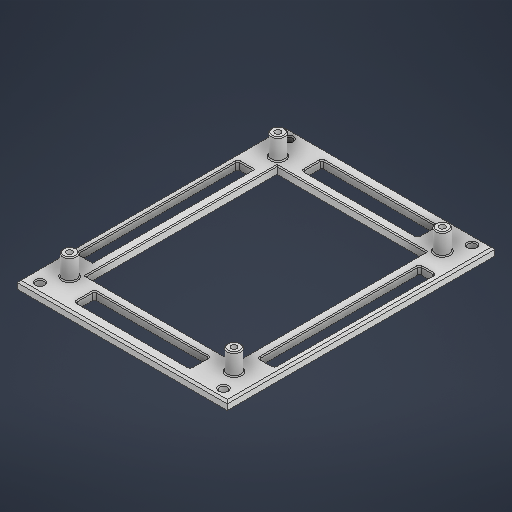
# Autodesk Inventor part: Base
Saved by Autodesk Inventor 2026 (Build 300175000, 175)
## iProperties
Created: 2026-02-15
Part Number: Base
Material: Generisch
Document SubType Name: Modeling
Designer: Jakob Dorninger
Density: 1 g/cm^3
Appearance: Vorgabe
Author: Jakob Dorninger
Autodesk Inventor part; units mm, degrees
ref_plane "YZ Plane" through (0, 0, 0) normal (1, 0, 0) x (0, 1, 0)
ref_plane "XZ Plane" through (0, 0, 0) normal (0, 1, 0) x (-1, 0, 0)
ref_plane "XY Plane" through (0, 0, 0) normal (0, 0, 1) x (1, 0, 0)
sketch "Skizze1" plane through (0, 0, 0) normal (0, 0, 1) x (1, 0, 0)
  line L0 (27.5, -35) -> (-27.5, -35)
  line L1 (-27.5, -35) -> (-27.5, 35)
  line L2 (-27.5, 35) -> (27.5, 35)
  line L3 (27.5, 35) -> (27.5, -35)
  line L4 (27.5, -35) -> (-27.5, 35) construction
  line L5 (-27.5, -35) -> (27.5, 35) construction
  line L6 (-19.5, -25) -> (19.5, -25)
  line L7 (19.5, -25) -> (19.5, 25)
  line L8 (19.5, 25) -> (-19.5, 25)
  line L9 (-19.5, 25) -> (-19.5, -25)
  line L10 (-19.5, -25) -> (19.5, 25) construction
  line L11 (19.5, -25) -> (-19.5, 25) construction
  point P0 (0, 0)
  dimension "d0" = 55
  dimension "d1" = 70
  dimension "d32" = 39
  dimension "d33" = 50
  constraints: 24 end point, 4 midpoint, 4 parallel, 2 horizontal, 2 perpendicular
  measures "d0" distance of L1.end L2.end
  measures "d1" distance of L0.end L1.end
  measures "d32" distance of L8.end L7.end
  measures "d33" distance of L7.end L6.end
extrude "Extrusion1" add sketch "Skizze1" along normal blind 2
sketch "Skizze2" plane through (0, 0, 2) normal (0, 0, 1) x (1, 0, 0)
  circle A0 centre (-21.5, 27.25) radius 1.75
  line L0 (0, -49) -> (0, 49) projected
  line L1 (-38.5, 0) -> (38.5, 0) projected
  circle A1 centre (-21.5, -27.25) radius 1.75
  circle A2 centre (21.5, 27.25) radius 1.75
  circle A3 centre (21.5, -27.25) radius 1.75
  point P0 (0, 0)
  dimension "d4" = 3.5
  dimension "d5" = 21.5
  dimension "d6" = 27.25
  dimension "d9" = 54.5
  dimension "d12" = 43
  constraints: 4 centre point, 1 horizontal, 1 vertical, 6 other
  measures "d4" diameter of A0
  measures "d5" horizontal distance of point (0, 0) A0.centre
  measures "d6" vertical distance of point (0, 0) A0.centre
  measures "d9" distance of A0.centre A1.centre
  measures "d12" distance of A0.centre A2.centre
extrude "Extrusion2" add sketch "Skizze2" along normal blind 5.5
sketch "Skizze3" plane through (-21.5, 27.25, 7.5) normal (0, 0, 1) x (1, 0, 0)
  circle A0 centre (0, 0) radius 1.75 projected
  line L0 (-17, -27.25) -> (60, -27.25) projected
  line L1 (21.5, -76.25) -> (21.5, 21.75) projected
  point P0 (21.5, -27.25)
  point P1 (0, -54.5)
  point P2 (43, 0)
  point P3 (43, -54.5)
  dimension "d19" = 54.5
  dimension "d22" = 43
  constraints: 1 coincident, 1 horizontal, 1 vertical, 3 other
  measures "d19" distance of point (0, 0) point (0, -54.5)
  measures "d22" distance of point (0, 0) point (43, 0)
hole "Bohrung1" at (-21.5, 27.25, 7.5) at (-21.5, -27.25, 7.5) at (21.5, 27.25, 7.5) at (21.5, -27.25, 7.5) direction (0, 0, -1) diameter 1.5 depth 5.5 tip angle 118
sketch "Skizze4" plane through (0, 0, 2) normal (0, 0, 1) x (1, 0, 0)
  line L0 (0, -49) -> (0, 49) projected
  line L1 (-38.5, 0) -> (38.5, 0) projected
  point P0 (0, 0)
  point P1 (-24, 32.5)
  point P2 (-24, -32.5)
  point P3 (24, 32.5)
  point P4 (24, -32.5)
  dimension "d34" = 24
  dimension "d35" = 32.5
  dimension "d38" = 65
  dimension "d41" = 48
  constraints: 1 horizontal, 1 vertical, 3 other
  measures "d34" horizontal distance of point (-24, 32.5) point (0, 0)
  measures "d35" vertical distance of point (0, 0) point (-24, 32.5)
  measures "d38" distance of point (-24, 32.5) point (-24, -32.5)
  measures "d41" distance of point (-24, 32.5) point (24, 32.5)
hole "Bohrung2" at (-24, 32.5, 2) at (-24, -32.5, 2) at (24, 32.5, 2) at (24, -32.5, 2) direction (0, 0, -1) diameter 2 depth 5.5 tip angle 118
chamfer "Fasen1" distance 0.5 angle 45 4 edges at (-27.5, 0, 2) (0, 35, 2) (27.5, 0, 2) (0, -35, 2)
chamfer "Fasen2" distance 0.25 angle 45 12 edges at (0, 25, 2) (-19.5, 0, 2) (0, -25, 2) (19.5, 0, 2) (19.75, 27.25, 7.5) (-23.25, 27.25, 7.5) (-23.25, -27.25, 7.5) (19.75, -27.25, 7.5) (-24, -31.5, 2) (24, -31.5, 2) (24, 33.5, 2) (-24, 33.5, 2)
sketch "Skizze5" plane through (0, 0, 2) normal (0, 0, 1) x (1, 0, 0)
  line L0 (-15, 32.25) -> (15, 32.25)
  line L1 (15, 32.25) -> (15, 27.25)
  line L2 (15, 27.25) -> (-15, 27.25)
  line L3 (-15, 27.25) -> (-15, 32.25)
  line L4 (-15, 32.25) -> (15, 27.25) construction
  line L5 (15, 32.25) -> (-15, 27.25) construction
  line L6 (-19.5, 25) -> (19.5, 25) projected
  line L7 (-38.5, 0) -> (38.5, 0) projected
  line L8 (0, -49) -> (0, 49) projected
  line L9 (-15, -32.25) -> (15, -32.25)
  line L10 (15, -32.25) -> (15, -27.25)
  line L11 (15, -27.25) -> (-15, -27.25)
  line L12 (-15, -27.25) -> (-15, -32.25)
  line L13 (25.75, -21) -> (21.75, -21)
  line L14 (21.75, -21) -> (21.75, 21)
  line L15 (21.75, 21) -> (25.75, 21)
  line L16 (25.75, 21) -> (25.75, -21)
  line L17 (25.75, -21) -> (21.75, 21) construction
  line L18 (21.75, -21) -> (25.75, 21) construction
  line L19 (27.5, -35) -> (27.5, 35) projected
  line L20 (-25.75, -21) -> (-21.75, -21)
  line L21 (-21.75, -21) -> (-21.75, 21)
  line L22 (-21.75, 21) -> (-25.75, 21)
  line L23 (-25.75, 21) -> (-25.75, -21)
  point P0 (0, 0)
  point P1 (0, 29.75)
  point P2 (23.75, 0)
  dimension "d57" = 4.75
  dimension "d58" = 30
  dimension "d59" = 5
  dimension "d60" = 3.75
  dimension "d61" = 4
  dimension "d62" = 42
  constraints: 40 end point, 8 symmetric about line, 4 midpoint, 4 parallel, 2 horizontal, 2 perpendicular, 1 point on line, 1 vertical alignment
  measures "d57" distance from line of L6 point (0, 29.75)
  measures "d58" distance of L1.end L2.end
  measures "d59" distance of L0.end L1.end
  measures "d60" distance from line of L19 point (23.75, 0)
  measures "d61" distance of L14.end L15.end
  measures "d62" distance of L15.end L13.start
extrude "Extrusion3" cut sketch "Skizze5" against normal through all
fillet "Rundung1" radius 0.5 14 edges at (15, 32.25, 1) (15, 27.25, 1) (25.75, 21, 1) (15, -27.25, 1) (-15, 32.25, 1) (-25.75, 21, 1) (21.75, 21, 1) (-15, 27.25, 1) (-25.75, -21, 1) (25.75, -21, 1) (15, -32.25, 1) (21.75, -21, 1) (-15, -27.25, 1) (-15, -32.25, 1)
chamfer "Fasen3" distance 0.25 angle 45 14 edges at (0, -32.25, 2) (-14.8536, -32.1036, 2) (-15, -29.75, 2) (-14.8536, -27.3964, 2) (0, -27.25, 2) (14.8536, -27.3964, 2) (15, -29.75, 2) (14.8536, -32.1036, 2) (-25.75, 0, 2) (-25.6036, 20.8536, 2) (-23.5, 21, 2) (-25.6036, -20.8536, 2) (-23.5, -21, 2) (-21.75, 0, 2)
chamfer "Fasen4" distance 0.25 angle 45 16 edges at (21.75, 0, 2) (21.8964, 20.8536, 2) (23.75, 21, 2) (25.6036, 20.8536, 2) (25.75, 0, 2) (25.6036, -20.8536, 2) (23.75, -21, 2) (21.8964, -20.8536, 2) (-15, 29.75, 2) (-14.8536, 32.1036, 2) (0, 32.25, 2) (14.8536, 32.1036, 2) (15, 29.75, 2) (14.8536, 27.3964, 2) (0, 27.25, 2) (-14.8536, 27.3964, 2)
fillet "Rundung2" radius 0.25 4 edges at (19.75, 27.25, 2) (-23.25, 27.25, 2) (-23.25, -27.25, 2) (19.75, -27.25, 2)
